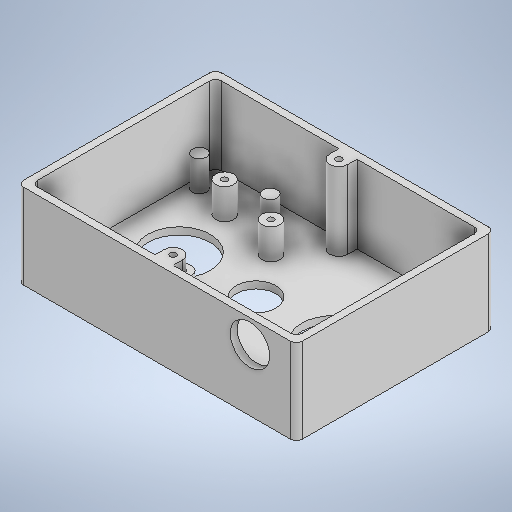
# Autodesk Inventor part: Box
Saved by Autodesk Inventor 2025 (Build 290162000, 162)
## iProperties
Created: 2024-06-08
Part Number: Box
Material: Generic
Document SubType Name: Modeling
Designer: Dell
Density: 1 g/cm^3
Appearance: Default
Author: Dell
Autodesk Inventor part; units mm, degrees
ref_plane "YZ Plane" through (0, 0, 0) normal (1, 0, 0) x (0, 1, 0)
ref_plane "XZ Plane" through (0, 0, 0) normal (0, 1, 0) x (-1, 0, 0)
sketch "Sketch1" plane through (0, 0, 0) normal (0, 1, 0) x (-1, 0, 0)
  line L0 (-66, 49) -> (66, 49)
  line L1 (69, 46) -> (69, -46)
  line L2 (66, -49) -> (-66, -49)
  line L3 (-69, -46) -> (-69, 46)
  line L4 (-69, 49) -> (69, -49) construction
  line L5 (69, 49) -> (-69, -49) construction
  arc A0 (69, 46) -> (66, 49) centre (66, 46) ccw
  arc A1 (-66, 49) -> (-69, 46) centre (-66, 46) ccw
  arc A2 (-69, -46) -> (-66, -49) centre (-66, -46) ccw
  arc A3 (66, -49) -> (69, -46) centre (66, -46) ccw
  line L6 (65.5, -42.5) -> (65.5, 42.5)
  line L7 (62.5, 45.5) -> (-62.5, 45.5)
  line L8 (-65.5, 42.5) -> (-65.5, -42.5)
  line L9 (-62.5, -45.5) -> (62.5, -45.5)
  arc A4 (65.5, 42.5) -> (62.5, 45.5) centre (62.5, 42.5) ccw
  arc A5 (-62.5, 45.5) -> (-65.5, 42.5) centre (-62.5, 42.5) ccw
  arc A6 (-65.5, -42.5) -> (-62.5, -45.5) centre (-62.5, -42.5) ccw
  arc A7 (62.5, -45.5) -> (65.5, -42.5) centre (62.5, -42.5) ccw
  point P0 (0, 0)
  dimension "d0" = 138
  dimension "d1" = 98
  dimension "d2" = 3
  dimension "d3" = 3.5
  dimension "d4" = 3
  constraints: 20 end point, 16 point on circle, 16 tangent, 8 centre point, 8 point on line, 6 equal radius, 4 parallel, 2 midpoint, 2 perpendicular, 1 horizontal, 3 other
  measures "d0" distance of L4.end L5.end
  measures "d1" distance of L5.start L4.end
  measures "d2" radius of A0
  measures "d3" distance between parallel lines of L1 L6
  measures "d4" radius of A4
extrude "Extrusion1" add sketch "Sketch1" along normal blind 3.5 contours A7 L9 A6 L8 A5 L7 A4 L6
extrude "Extrusion2" add sketch "Sketch1" along normal blind 42
sketch "Sketch2" plane through (0, 3.5, 0) normal (0, 1, 0) x (1, 0, 0)
  circle A0 centre (-14.4905, 21.8769) radius 1.5
  line L0 (-17.4775, 25.0064) -> (63, 25.0064)
  line L1 (-17.4775, -25.0064) -> (-17.4775, 25.0064)
  circle A1 centre (-14.4905, -22.0231) radius 1.5
  line L2 (63, -25.0064) -> (-17.4775, -25.0064)
  circle A2 centre (60.3095, -22.0231) radius 1.5
  line L3 (63, 25.0064) -> (63, -25.0064)
  circle A3 centre (60.3095, 21.8769) radius 1.5
  line L4 (-62.5, -45.5) -> (62.5, -45.5) projected
  circle A4 centre (-14.4905, -22.0231) radius 4.5
  circle A5 centre (-14.4905, 21.8769) radius 4.5
  circle A6 centre (60.3095, 21.8769) radius 4.5
  circle A7 centre (60.3095, -22.0231) radius 4.5
  arc A8 (-65.5, -42.5) -> (-62.5, -45.5) centre (-62.5, -42.5) ccw projected
  line L5 (-62.5, -45.5) -> (62.5, -45.5) projected
  arc A9 (62.5, -45.5) -> (65.5, -42.5) centre (62.5, -42.5) ccw projected
  line L6 (65.5, -42.5) -> (65.5, 42.5) projected
  arc A10 (65.5, 42.5) -> (62.5, 45.5) centre (62.5, 42.5) ccw projected
  line L7 (62.5, 45.5) -> (-62.5, 45.5) projected
  arc A11 (-62.5, 45.5) -> (-65.5, 42.5) centre (-62.5, 42.5) ccw projected
  line L8 (-65.5, 42.5) -> (-65.5, -42.5) projected
  line L9 (-65.5, -42.5) -> (-65.5, 42.5) projected
  line L10 (-65.5, 0) -> (-27.8028, 0)
  point P0 (0, 0)
  point P1 (22.7612, -25.0064)
  point P2 (-17.4775, 0)
  dimension "d9" = 3
  dimension "d10" = 80.4775
  dimension "d11" = 50.0127
  dimension "d14" = 2.6905
  dimension "d15" = 46.8833
  dimension "d16" = 2.6905
  dimension "d17" = 2.9833
  dimension "d18" = 77.4905
  dimension "d19" = 46.8833
  dimension "d20" = 77.4905
  dimension "d21" = 2.9833
  dimension "d23" = 9
  dimension "d24" = 9
  dimension "d25" = 9
  dimension "d26" = 9
  dimension "d59" = 2.5
  constraints: 10 end point, 8 centre point, 4 coincident, 3 equal radius, 3 midpoint, 2 horizontal, 2 parallel, 1 point on line, 1 vertical
  measures "d9" diameter of A3
  measures "d10" distance between parallel lines of L3 L1
  measures "d11" distance between parallel lines of L2 L0
  measures "d14" distance from line of A3.centre L3
  measures "d15" distance from line of A3.centre L2
  measures "d16" distance from line of A2.centre L3
  measures "d17" distance from line of A2.centre L2
  measures "d18" distance from line of A0.centre L3
  measures "d19" distance from line of A0.centre L2
  measures "d20" distance from line of A1.centre L3
  measures "d21" distance from line of A1.centre L2
  measures "d23" diameter of A4
  measures "d24" diameter of A5
  measures "d25" diameter of A6
  measures "d26" diameter of A7
  measures "d59" distance between parallel lines of L3 L6
extrude "Extrusion3" add sketch "Sketch2" along normal blind 15 contours L1 A5 L0 | L0 A5 L1 | A6 L3 L0 | L0 L3 A6 | A4 L2 L1 | L1 L2 A4 | A7 L2 L3 | L3 L2 A7
sketch "Sketch4" plane through (0, 3.5, 0) normal (0, 1, 0) x (1, 0, 0)
  circle A0 centre (-43.1118, 27.6225) radius 1.5
  circle A1 centre (-43.1118, -27.6225) radius 1.5
  circle A2 centre (-25.6112, -27.6225) radius 1.4605
  circle A3 centre (-60.6124, 27.6225) radius 1.4605
  line L0 (-30.3737, -42.9768) -> (-36.7237, -42.9768)
  line L1 (-55.8383, 42.9768) -> (-49.4883, 42.9768)
  line L2 (-23.2236, -13.1064) -> (-23.2236, 13.1572)
  line L3 (-63, 13.1572) -> (-63, -13.1064)
  line L4 (-65.5, 42.5) -> (-65.5, -42.5) projected
  line L5 (-65.5, 0) -> (-9.8345, 0)
  line L6 (-43.1118, -27.6225) -> (-43.1118, 27.6225)
  circle A4 centre (-60.6124, -27.6225) radius 1.4605
  circle A5 centre (-25.6112, 27.6225) radius 1.4605
  circle A6 centre (-60.6124, 32.6225) radius 3.5
  circle A7 centre (-60.6124, -32.6225) radius 3.5
  circle A8 centre (-25.6112, 32.6225) radius 3.5
  circle A9 centre (-25.6112, -32.6225) radius 3.5
  circle A10 centre (-43.1118, -27.6225) radius 4.5
  circle A11 centre (-43.1118, 27.6225) radius 4.5
  point P0 (0, 0)
  point P1 (-43.1997, -2.4081)
  point P2 (-43.1118, 0)
  dimension "d35" = 2.921
  dimension "d36" = 3
  dimension "d37" = 39.7764
  dimension "d38" = 85.9536
  dimension "d41" = 56.134
  dimension "d42" = 29.8704
  dimension "d43" = 2.3876
  dimension "d44" = 15.3543
  dimension "d45" = 7.1501
  dimension "d46" = 13.5001
  dimension "d47" = 19.8882
  dimension "d48" = 70.5993
  dimension "d49" = 19.8882
  dimension "d50" = 15.3543
  dimension "d51" = 19.9761
  dimension "d52" = 40.5687
  dimension "d53" = 26.2647
  dimension "d54" = 32.6147
  dimension "d55" = 37.3888
  dimension "d56" = 70.5993
  dimension "d57" = 56.134
  dimension "d58" = 29.8704
  dimension "d60" = 2.5
  dimension "d61" = 7
  dimension "d62" = 5
  dimension "d63" = 9
  dimension "d64" = 9
  constraints: 12 centre point, 12 end point, 5 symmetric about line, 2 coincident, 2 equal radius, 2 horizontal, 2 midpoint, 2 parallel, 1 point on line, 1 vertical, 5 other
  measures "d35" diameter of A2
  measures "d36" diameter of A0
  measures "d37" distance between parallel lines of L2 L3
  measures "d38" distance between parallel lines of L0 L1
  measures "d41" distance from line of L2.end L0
  measures "d42" distance from line of L2.start L0
  measures "d43" distance from line of A2.centre L2
  measures "d44" distance from line of A2.centre L0
  measures "d45" distance from line of L0.start L2
  measures "d46" distance from line of L0.end L2
  measures "d47" distance from line of L6.end L2
  measures "d48" distance from line of L6.end L0
  measures "d49" distance from line of L6.start L2
  measures "d50" distance from line of L6.start L0
  measures "d51" distance from line of point (-43.2, -2.408) L2
  measures "d52" distance from line of point (-43.2, -2.408) L0
  measures "d53" distance from line of L1.end L2
  measures "d54" distance from line of L1.start L2
  measures "d55" distance from line of A3.centre L2
  measures "d56" distance from line of A3.centre L0
  measures "d57" distance from line of L3.start L0
  measures "d58" distance from line of L3.end L0
  measures "d60" distance between parallel lines of L4 L3
  measures "d61" diameter of A6
  measures "d62" distance of A6.centre A3.centre
  measures "d63" diameter of A10
  measures "d64" diameter of A11
extrude "Extrusion5" add sketch "Sketch4" along normal blind 15 contours A11 | A10 | A6 | A7 | A8 | A9
sketch "Sketch5" plane through (0, 3.5, 0) normal (0, 1, 0) x (1, 0, 0)
  circle A0 centre (0, 0) radius 9.75
  circle A1 centre (38.1, 0) radius 15.5
  circle A2 centre (-38.1, 0) radius 15.5
  dimension "d67" = 19.5
  dimension "d68" = 31
  dimension "d69" = 31
  dimension "d70" = 38.1
  dimension "d71" = 38.1
  constraints: 3 centre point, 1 coincident
  measures "d67" diameter of A0
  measures "d68" diameter of A1
  measures "d69" diameter of A2
  measures "d70" distance of A1.centre point (0, 0)
  measures "d71" distance of A2.centre point (0, 0)
extrude "Extrusion6" cut sketch "Sketch5" against normal through all
ref_plane "Work Plane1" through (0, 0, 46) normal (1, 0, 0) x (0, 0, -1)
sketch "Sketch8" plane through (62.5, 3.5, 45.5) normal (0, 0, -1) x (-1, 0, 0)
  line L0 (-6.5, -3.5) -> (-6.5, 38.5) projected
  line L1 (6.6905, 15) -> (-2.3095, 15) projected
  circle A0 centre (16.5, 27) radius 9.75
  line L2 (0, 0) -> (0, 38.5) projected
  point P0 (62.5, -3.5)
  dimension "d83" = 19.5
  dimension "d84" = 12
  dimension "d87" = 16.5
  constraints: 1 centre point
  measures "d83" diameter of A0
  measures "d84" distance from line of A0.centre L1
  measures "d87" distance from line of L2 A0.centre
extrude "Extrusion8" cut sketch "Sketch8" against normal through all
sketch "Sketch9" plane through (0, 3.5, 0) normal (0, 1, 0) x (1, 0, 0)
  circle A0 centre (0, -41) radius 1.5
  circle A1 centre (0, -41) radius 4.5
  line L0 (62.5, -45.5) -> (-62.5, -45.5) projected
  line L1 (-4.5, -41) -> (-4.5, -45.5)
  line L2 (4.5, -41) -> (4.5, -45.5)
  line L3 (-65.5, -42.5) -> (-65.5, 42.5) projected
  line L4 (-65.5, 0) -> (0, 0)
  circle A2 centre (0, 41) radius 1.5
  circle A3 centre (0, 41) radius 4.5
  line L5 (-4.5, 41) -> (-4.5, 45.5)
  line L6 (4.5, 41) -> (4.5, 45.5)
  line L7 (-62.5, 45.5) -> (62.5, 45.5) projected
  dimension "d88" = 3
  dimension "d89" = 9
  dimension "d90" = 4.5
  constraints: 10 end point, 6 symmetric about line, 4 centre point, 4 point on circle, 2 coincident, 2 perpendicular, 2 point on line, 1 horizontal, 1 midpoint, 1 tangent, 2 other
  measures "d88" diameter of A0
  measures "d89" diameter of A1
  measures "d90" distance from line of L0 A0.centre
extrude "Extrusion9" add sketch "Sketch9" along normal up to surface (38.5 mm away)
equation "\"d0\" = BoxL"
equation "\"d1\" = BoxW"
equation "\"d2\" = BoxCorner"
equation "\"d3\" = BoxWall"
equation "\"d4\" = BoxCorner"
equation "\"d7\" = BoxH"
equation "\"BoxW\" = 98"
equation "\"BoxL\" = 138"
equation "\"BoxCorner\" = 3"
equation "\"BoxWall\" = 3.5"
equation "\"BoxH\" = 42"
equation "\"PinH\" = 15"
body "Solid1"
